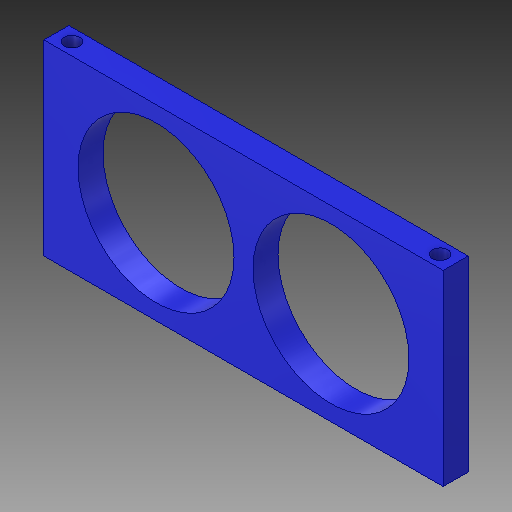
# Autodesk Inventor part: Separator1
Saved by Autodesk Inventor 2019.2 (Build 232265000, 265)
## iProperties
Created: 2018-09-25
Part Number: Separator1
Material: Generic
Document SubType Name: Modeling
Designer: eroldan
Density: 1 g/cm^3
Appearance: Default
Author: eroldan
Autodesk Inventor part; units mm, degrees
ref_plane "YZ Plane" through (0, 0, 0) normal (1, 0, 0) x (0, 1, 0)
ref_plane "XZ Plane" through (0, 0, 0) normal (0, 1, 0) x (-1, 0, 0)
ref_plane "XY Plane" through (0, 0, 0) normal (0, 0, 1) x (1, 0, 0)
sketch "Sketch1" plane through (0, 0, 0) normal (0, 0, 1) x (1, 0, 0)
  line L0 (-64, -30) -> (64, -30)
  line L1 (64, -30) -> (64, 30)
  line L2 (64, 30) -> (-64, 30)
  line L3 (-64, 30) -> (-64, -30)
  line L4 (-64, -30) -> (64, 30) construction
  line L5 (64, -30) -> (-64, 30) construction
  point P0 (0, 0)
  dimension "d0" = 128
  dimension "d1" = 60
  constraints: 12 end point, 2 midpoint, 2 parallel, 1 horizontal, 1 perpendicular
  measures "d0" distance of L2.end L1.end
  measures "d1" distance of L1.end L0.end
extrude "Extrusion1" add sketch "Sketch1" along normal blind 8
sketch "Sketch2" plane through (-64, 30, 0) normal (0, 1, 0) x (1, 0, 0)
  line L0 (128, 0) -> (0, 0) projected
  line L1 (0, 0) -> (0, -8) projected
  line L2 (128, -8) -> (0, -8) projected
  line L3 (128, 0) -> (128, -8) projected
  point P0 (64, 0)
  point P1 (5, -4)
  point P2 (123, -4)
  dimension "d4" = 5
  dimension "d5" = 5
  measures "d4" distance from line of L1 point (5, -4)
  measures "d5" distance from line of L3 point (123, -4)
hole "Hole1" at (-59, 30, 4) at (59, 30, 4) direction (0, -1, 0) diameter 5 end through all
sketch "Sketch3" plane through (-64, -30, 0) normal (0, -1, 0) x (1, 0, 0)
  point P0 (64, 0)
sketch "Sketch4" plane through (0, 0, 0) normal (0, 0, -1) x (-1, 0, 0)
  line L0 (0, 0) -> (0, 24.6794) construction
  point P0 (-28.0484, 0)
  point P1 (28.0484, 0)
  constraints: 2 end point, 1 symmetric about line, 1 vertical
hole "Hole2" at (-28.0484, 0, 0) at (28.0484, 0, 0) direction (0, 0, 1) diameter 50 end through all
equation "\"d5\" = d4"
body "Solid1"
